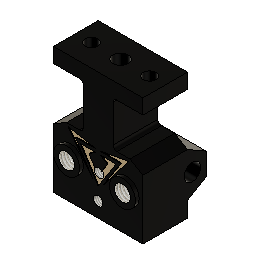
V2 Mothend (Autodesk Fusion 360 design; units mm, degrees)
part number: V2 Mothend BETA
Autodesk Fusion 360 part; units mm, degrees
ref_plane "WorkPlane1" through (0, 0, 3.5) normal (0, 0, 1) x (1, 0, 0) in component "Mothblock"
sketch "Sketch1" plane through (0, 0, 3.5) normal (0, 0, 1) x (0, 1, 0) in component "Mothblock"
  circle A0 centre (0, 0) radius 3.5
  line L0 (6, -12) -> (-6, -12)
  line L1 (-6, -12) -> (-6, 12)
  line L2 (-6, 12) -> (6, 12)
  line L3 (6, 12) -> (6, -12)
  line L4 (6, -12) -> (-6, 12) construction
  line L5 (-6, -12) -> (6, 12) construction
  line L6 (0, 7) -> (0, -7) construction
  line L7 (-3.75, 7.5) -> (3.75, 7.5) construction
  line L8 (3.75, 7.5) -> (3.75, -7.5) construction
  line L9 (3.75, -7.5) -> (-3.75, -7.5) construction
  line L10 (-3.75, -7.5) -> (-3.75, 7.5) construction
  line L11 (-3.75, 7.5) -> (3.75, -7.5) construction
  line L12 (3.75, 7.5) -> (-3.75, -7.5) construction
  dimension "d90" = 7
  dimension "d346" = 12
  dimension "d347" = 24
  dimension "d350" = 14
  dimension "d563" = 15
  dimension "d564" = 7.5
  constraint coincident A0.centre origin
  constraint horizontal L0
  constraint perpendicular L0 L1
  constraint parallel L0 L2
  constraint parallel L1 L3
  constraint coincident L4 A0.centre
  constraint coincident L5 A0.centre
  constraint vertical L6
  constraint midpoint A0.centre L6
  constraint horizontal L7
  constraint perpendicular L7 L8
  constraint parallel L7 L9
  constraint parallel L8 L10
  constraint coincident L11 A0.centre
  constraint coincident L12 A0.centre
  measures "d90" diameter of A0
  measures "d346" distance of L1.end L2.end
  measures "d347" distance of L0.end L1.end
  measures "d350" distance of L6.start L6.end
  measures "d563" distance of L7.end L8.end
  measures "d564" distance of L7.start L7.end
extrude "Extrude1" add sketch "Sketch1" along normal blind 34 contours A0 | L0 L1 L2 L3 in component "Mothblock"
hole "Hole8" [suppressed] in component "Mothblock"
thread "Thread9" [suppressed] in component "Mothblock"
hole "Hole15" at (-7.5, 3.75, 3.5) at (-7.5, -3.75, 3.5) at (7.5, 3.75, 3.5) at (7.5, -3.75, 3.5) direction (0, 0, 1) diameter 2.45 depth 6 tip angle 118 in component "Mothblock"
hole "Hole21" at (0, 0, 3.5) direction (0, 0, 1) diameter 4.1 end through all counterbore diameter 7.15 counterbore depth 14.5 in component "Mothblock"
sketch "Sketch7" plane through (0, -6, 0) normal (0, -1, 0) x (1, 0, 0) in component "Mothblock"
  line L0 (0, 3.5) -> (0, 37.5)
  line L1 (-12, 19.5) -> (-4, 24.1188)
  line L2 (-4, 24.1188) -> (-4, 33.5)
  line L3 (-12, 3.5) -> (12, 3.5)
  line L4 (12, 3.5) -> (12, 37.5)
  line L5 (12, 37.5) -> (-12, 37.5)
  line L6 (-12, 37.5) -> (-12, 3.5)
  line L7 (-4, 33.5) -> (-12, 33.5)
  line L8 (12, 19.5) -> (4, 24.1188)
  line L9 (4, 24.1188) -> (4, 33.5)
  line L10 (4, 33.5) -> (12, 33.5)
  line L11 (-8.5, 21.5207) -> (-4, 21.5207)
  line L12 (-4, 21.5207) -> (-4, 24.1188)
  line L13 (8.5, 21.5207) -> (4, 21.5207)
  line L14 (4, 21.5207) -> (4, 24.1188)
  line L15 (-6.25, 21.5207) -> (-4, 22.8198)
  line L16 (6.25, 21.5207) -> (4, 22.8198)
  dimension "d403" = 4
  dimension "d404" = 16
  dimension "d405" = 60
  dimension "d406" = 8
  dimension "d408" = 8
  dimension "d594" = 3.5
  dimension "d616" = 8
  dimension "d617" = 4.5
  dimension "d650" = 11.9793
  constraint vertical L0
  constraint symmetric L0 L1.start L8.start
  constraint symmetric L0 L1.end L8.end
  constraint symmetric L0 L2.end L9.end
  constraint symmetric L0 L7.end L10.end
  constraint coincident L6 L7.end
  constraint coincident L1.start L6
  constraint midpoint L0.start L3
  constraint horizontal L7
  constraint perpendicular L9 L10
  constraint midpoint L0.end L5
  constraint perpendicular L0 L11
  constraint coincident L1.end L2.start
  constraint perpendicular L11 L12
  constraint symmetric L0 L11.start L13.start
  constraint symmetric L0 L11.end L13.end
  constraint coincident L1 L11.start
  constraint midpoint L11 L15.start
  constraint coincident L12 L15.end
  constraint parallel L1 L15
  constraint symmetric L0 L15.start L16.start
  constraint symmetric L0 L15.end L16.end
  measures "d403" distance of L5.end L7.end
  measures "d404" distance of L1.start L3.start
  measures "d405" angle of L1 L6
  measures "d406" distance of L2 L9
  measures "d408" distance of L9.end L10.end
  measures "d594" horizontal distance of L1.start L11.start
  measures "d616" distance of L2.end L7.end
  measures "d617" distance of L11.start L11.end
  measures "d650" distance of L7 L11.start
extrude "Extrude7" cut sketch "Sketch7" against normal through all contours L1 L2 L6 L7 | L4 L8 L9 L10 | L1 L11 L12 L15 | L8 L13 L14 L16 | L11 L12 L15 | L13 L14 L16 in component "Mothblock"
sketch "Sketch2" plane through (0, 0, 37.5) normal (0, 0, 1) x (1, 0, 0) in component "Mothblock"
  circle A0 centre (0, 0) radius 2.05
  circle A1 centre (7.8, 0) radius 1.6
  circle A2 centre (-7.8, 0) radius 1.6
  line L0 (-7.8, 0) -> (7.8, 0) construction
  line L1 (-12, 6) -> (-12, -6)
  line L2 (-12, -6) -> (12, -6)
  line L3 (12, -6) -> (12, 6)
  line L4 (12, 6) -> (-12, 6)
  line L5 (-12, 6) -> (-4, 6)
  line L6 (-4, 6) -> (-4, -6)
  line L7 (-4, -6) -> (-12, -6)
  line L8 (-12, -6) -> (-12, 6)
  line L9 (-7.8, 6) -> (-7.8, -6) construction
  circle A3 centre (0, 0) radius 2.05
  dimension "d71" = 4.1
  dimension "d72" = 3.2
  dimension "d73" = 15.6
  constraint coincident A2.centre L0.start
  constraint coincident A1.centre L0.end
  constraint midpoint A0.centre L0
  constraint equal A1 A2
  constraint coincident A0.centre A3.centre
  constraint horizontal L0
  constraint coincident A2.centre L9
  constraint coincident L2 L9.end
  constraint coincident L4 L9.start
  constraint perpendicular L5 L9
  measures "d71" diameter of A0
  measures "d72" diameter of A1
  measures "d73" distance of A1.centre A2.centre
hole "Hole14" at (-7.8, 0, 37.5) at (7.8, 0, 37.5) direction (0, 0, -1) diameter 3.4 end up to surface (4 mm away) in component "Mothblock"
fillet "Fillet1" radius 1 4 edges at (4, 0, 21.5207) (-4, 0, 21.5207) (4, 0, 33.5) (-4, 0, 33.5) in component "Mothblock"
sketch "Sketch3" plane through (12, 0, 0) normal (-1, 0, 0) x (0, 1, 0) in component "Mothblock"
  line L0 (11, -16.6132) -> (11, -10.6132)
  line L1 (0, -3.5) -> (0, -19.5) construction
  line L2 (11, -16.6132) -> (6, -19.5)
  line L3 (11, -13.6132) -> (6, -13.6132) construction
  circle A0 centre (7.3175, -13.6132) radius 2.2425 construction
  line L4 (11, -10.6132) -> (6, -7.7265)
  line L5 (-3.5, -3.5) -> (3.5, -3.5)
  line L6 (6, -19.5) -> (-6, -19.5) construction
  line L7 (-6, -19.5) -> (-6, -3.5) construction
  line L8 (-6, -3.5) -> (6, -3.5) construction
  line L9 (6, -3.5) -> (6, -19.5) construction
  line L10 (-3.575, -3.5) -> (3.575, -3.5)
  line L11 (-3.575, -18) -> (3.575, -18)
  line L12 (3.575, -18) -> (3.575, -3.5) construction
  line L13 (6, -19.5) -> (6, -7.7265)
  dimension "d145" = 6
  dimension "d415" = 4.485
  dimension "d573" = 5
  dimension "d574" = 60
  dimension "d575" = 1.5
  dimension "d626" = 1.44
  dimension "d644" = 13.3175
  dimension "d645" = 10.1132
  constraint vertical L0
  constraint midpoint L0 L3.start
  constraint coincident L3 A0.centre
  constraint symmetric L0.start L3 L0.end
  constraint symmetric L3 L4.end L2.end
  constraint midpoint L1.end L6
  constraint midpoint L1.start L5
  constraint coincident L3.end L9
  constraint coincident L2.end L6.start
  constraint coincident L4.end L9
  constraint perpendicular L3 L9
  constraint coincident L11.end L12.start
  constraint coincident L10.end L12.end
  measures "d145" distance of L0.start L0.end
  measures "d415" diameter of A0
  measures "d573" horizontal distance of L3.start L3.end
  measures "d574" angle of L4 L9
  measures "d575" distance of A0 L12
  measures "d626" distance of L0 A0
  measures "d644" horizontal distance of A0.centre L7.end
  measures "d645" vertical distance of A0.centre L8.end
extrude "Extrude11" add sketch "Sketch3" along normal up to surface (24 mm away) in component "Mothblock"
hole "Hole13" at (12, 7.3175, 13.6132) direction (-1, 0, 0) diameter 4.4 depth 22 tip angle 180 in component "Mothblock"
sketch "Sketch16" plane through (12, 0, 0) normal (1, 0, 0) x (0, 1, 0) in component "Mothblock"
  circle A0 centre (7.3175, 13.6132) radius 2.2
  line L0 (6, 19.5) -> (-6, 19.5)
  line L1 (-6, 19.5) -> (-6, 3.5)
  line L2 (-6, 3.5) -> (6, 3.5)
  line L3 (6, 3.5) -> (6, 7.7265)
  line L4 (6, 7.7265) -> (11, 10.6132)
  line L5 (11, 10.6132) -> (11, 16.6132)
  line L6 (11, 16.6132) -> (6, 19.5)
  circle A1 centre (7.3175, 13.6132) radius 2.2
hole "Hole22" at (12, 7.3175, 13.6132) direction (-1, 0, 0) diameter 4.485 depth 3 tip angle 118 in component "Mothblock"
sketch "Sketch10" plane through (0, -6, 0) normal (0, 1, 0) x (-1, 0, 0) in component "Mothblock"
  line L0 (0, 0) -> (0, 3.5)
  line L1 (10, 13.6132) -> (0, 13.6132) construction
  line L2 (-3.575, 18) -> (-3.575, 3.5) construction
  line L3 (3.5, 27.2) -> (3.5, 14.2) construction
  line L4 (10, 15.8132) -> (-12, 15.8132) construction
  line L5 (10, 11.4132) -> (-12, 11.4132) construction
  circle A0 centre (-7.5, 13.6132) radius 2.5
  circle A1 centre (7.5, 13.6132) radius 2.5
  line L6 (-6.3895, 3.5) -> (-7.6105, 3.5)
  circle A2 centre (0, 14) radius 1.5
  circle A3 centre (0, 7.5) radius 1.5
  line L7 (-6.3895, 9.5) -> (-7.6105, 9.5)
  line L8 (-6.3, 3.5) -> (-8.7, 3.5)
  line L9 (-6.3, 9.5) -> (-8.7, 9.5)
  line L10 (12, 33.5) -> (5, 33.5)
  line L11 (4, 32.5) -> (4, 22.5207)
  line L12 (5, 21.5207) -> (8.5, 21.5207)
  line L13 (8.5, 21.5207) -> (12, 19.5)
  line L14 (12, 19.5) -> (12, 3.5)
  line L15 (12, 3.5) -> (-12, 3.5)
  line L16 (-12, 3.5) -> (-12, 19.5)
  line L17 (-12, 19.5) -> (-8.5, 21.5207)
  line L18 (-8.5, 21.5207) -> (-5, 21.5207)
  line L19 (-4, 22.5207) -> (-4, 32.5)
  line L20 (-5, 33.5) -> (-12, 33.5)
  line L21 (-12, 33.5) -> (-12, 37.5)
  line L22 (-12, 37.5) -> (12, 37.5)
  line L23 (12, 37.5) -> (12, 33.5)
  line L24 (10, 11.4132) -> (10, 15.8132)
  line L25 (3.575, 3.5) -> (-3.575, 3.5)
  line L26 (3.575, 18) -> (-3.575, 18)
  line L27 (-3.575, 10.75) -> (4.0823, 10.75) construction
  arc A4 (5, 33.5) -> (4, 32.5) centre (5, 32.5) ccw
  arc A5 (4, 22.5207) -> (5, 21.5207) centre (5, 22.5207) ccw
  arc A6 (-5, 21.5207) -> (-4, 22.5207) centre (-5, 22.5207) ccw
  arc A7 (-4, 32.5) -> (-5, 33.5) centre (-5, 32.5) ccw
  line L28 (-8.9745, 15.8132) -> (-8.9745, 11.4132)
  dimension "d370" = 5
  dimension "d371" = 15
  dimension "d383" = 3
  dimension "d385" = 3
  dimension "d429" = 1.5
  dimension "d593" = 4
  constraint coincident L0.start origin
  constraint coincident L0 L1.end
  constraint perpendicular L0 L1
  constraint symmetric L0 A0 A1
  constraint coincident L1 A0.centre
  constraint coincident L0 A2.centre
  constraint coincident L0 A3.centre
  constraint horizontal L4
  constraint horizontal L5
  constraint midpoint L1.start L24
  constraint coincident L2.start L26.end
  constraint coincident L2.end L15
  constraint coincident L2.end L25.end
  constraint coincident L4.start L24.end
  constraint coincident L5.start L24.start
  constraint midpoint L2 L27.start
  constraint perpendicular L2 L27
  constraint symmetric A2.centre A3.centre L27
  measures "d370" diameter of A0
  measures "d383" diameter of A2
  measures "d385" diameter of A3
  measures "d429" distance of L3 A1
  measures "d593" distance of A2.centre L26
hole "Hole17" at (7.5, -6, 13.6132) at (-7.5, -6, 13.6132) direction (0, 1, 0) diameter 4.234 depth 13.25 tip angle 180 in component "Mothblock"
thread "Thread20" "ISO Metric profile 5.0 M5x0.8 M5x0.8 6H" thread offset 0 thread depth 7.4 in component "Mothblock"
hole "Hole18" at (0, -6, 7.5) at (0, -6, 14) direction (0, 1, 0) diameter 2.529 depth 6 tip angle 180 in component "Mothblock"
thread "Thread17" "ISO Metric profile 3.0 M3x0.5 M3x0.5 6H" major diameter 3.086 minor diameter 2.529 pitch 0.5 angle 60 resizes the face on face at (-1.2645, -5.1146, 7.505) on face at (-1.2645, -5.1146, 14.005) in component "Mothblock"
sketch "Sketch12" plane through (0, -6, 0) normal (0, -1, 0) x (1, 0, 0) in component "Mothblock"
  circle A0 centre (0, 7.5) radius 1.2645
  circle A1 centre (0, 14) radius 1.2645
  circle A2 centre (7.5, 13.6132) radius 2.117
  circle A3 centre (-7.5, 13.6132) radius 2.117
  line L0 (-12, 33.5) -> (-5, 33.5)
  line L1 (-4, 32.5) -> (-4, 22.5207)
  line L2 (-5, 21.5207) -> (-8.5, 21.5207)
  line L3 (-8.5, 21.5207) -> (-12, 19.5)
  line L4 (-12, 19.5) -> (-12, 3.5)
  line L5 (-12, 3.5) -> (12, 3.5)
  line L6 (12, 3.5) -> (12, 19.5)
  line L7 (12, 19.5) -> (8.5, 21.5207)
  line L8 (8.5, 21.5207) -> (5, 21.5207)
  line L9 (4, 22.5207) -> (4, 32.5)
  line L10 (5, 33.5) -> (12, 33.5)
  line L11 (12, 33.5) -> (12, 37.5)
  line L12 (12, 37.5) -> (-12, 37.5)
  line L13 (-12, 37.5) -> (-12, 33.5)
  circle A4 centre (7.5, 13.6132) radius 2.117
  circle A5 centre (-7.5, 13.6132) radius 2.117
  circle A6 centre (7.5, 13.6132) radius 3.5
  circle A7 centre (-7.5, 13.6132) radius 3.5
  arc A8 (-4, 32.5) -> (-5, 33.5) centre (-5, 32.5) ccw
  arc A9 (-5, 21.5207) -> (-4, 22.5207) centre (-5, 22.5207) ccw
  arc A10 (4, 22.5207) -> (5, 21.5207) centre (5, 22.5207) ccw
  arc A11 (5, 33.5) -> (4, 32.5) centre (5, 32.5) ccw
  dimension "d624" = 7
  dimension "d625" = 1.383
  constraint equal A6 A7
  measures "d624" diameter of A6
  measures "d625" distance of A4 A6
extrude "Extrude20" add sketch "Sketch12" along normal blind 1 contours A6 | A7 in component "Mothblock"
sketch "Sketch14" plane through (0, -6, 0) normal (0, -1, 0) x (1, 0, 0) in component "Mothblock"
  spline S0 degree 3 poles (0.0304, 11.0848) (0.0854, 11.1563) (0.5074, 11.7942) (0.7506, 12.1736) knots 0 0 0 0 1 1 1 1
  spline S1 degree 3 poles (0.7506, 12.1736) (0.8585, 12.342) (1.1188, 12.749) (1.329, 13.0781) knots 0 0 0 0 1 1 1 1
  spline S2 degree 3 poles (1.329, 13.0781) (1.8478, 13.8905) (2.3833, 14.7224) (2.905, 15.5267) knots 0 0 0 0 1 1 1 1
  spline S3 degree 3 poles (2.905, 15.5267) (4.115, 17.3924) (4.6109, 18.1742) (4.6967, 18.3521) knots 0 0 0 0 1 1 1 1
  spline S4 degree 3 poles (4.6967, 18.3521) (4.7099, 18.3795) (4.7145, 18.3987) (4.709, 18.4042) knots 0 0 0 0 1 1 1 1
  spline S5 degree 3 poles (4.709, 18.4042) (4.6779, 18.4351) (3.4737, 18.479) (1.9183, 18.5058) knots 0 0 0 0 1 1 1 1
  spline S6 degree 3 poles (1.9183, 18.5058) (1.2764, 18.5169) (0.6185, 18.515) (0.6057, 18.5019) knots 0 0 0 0 1 1 1 1
  spline S7 degree 3 poles (0.6057, 18.5019) (0.5804, 18.4762) (0.8663, 18.2891) (1.6579, 17.8133) knots 0 0 0 0 1 1 1 1
  spline S8 degree 3 poles (1.6579, 17.8133) (2.2194, 17.4758) (2.4139, 17.3559) (2.4225, 17.342) knots 0 0 0 0 1 1 1 1
  spline S9 degree 3 poles (2.4225, 17.342) (2.4529, 17.2928) (2.2808, 17.0041) (1.626, 16.0063) knots 0 0 0 0 1 1 1 1
  spline S10 degree 3 poles (1.626, 16.0063) (1.2373, 15.4139) (0.8859, 14.8661) (0.4954, 14.2436) knots 0 0 0 0 1 1 1 1
  spline S11 degree 3 poles (0.4954, 14.2436) (0.2267, 13.8154) (0.1401, 13.687) (0.0731, 13.6176) knots 0 0 0 0 1 1 1 1
  spline S12 degree 3 poles (0.0731, 13.6176) (-0.0446, 13.4956) (-0.0998, 13.5241) (-0.2628, 13.7908) knots 0 0 0 0 1 1 1 1
  spline S13 degree 3 poles (-0.2628, 13.7908) (-0.4707, 14.131) (-0.9331, 14.855) (-1.494, 15.7185) knots 0 0 0 0 1 1 1 1
  spline S14 degree 3 poles (-1.494, 15.7185) (-1.9472, 16.4162) (-2.1645, 16.7582) (-2.3415, 17.0518) knots 0 0 0 0 1 1 1 1
  spline S15 degree 3 poles (-2.3415, 17.0518) (-2.4493, 17.2307) (-2.4791, 17.2878) (-2.473, 17.3037) knots 0 0 0 0 1 1 1 1
  spline S16 degree 3 poles (-2.473, 17.3037) (-2.4671, 17.3191) (-2.3512, 17.4068) (-2.2296, 17.4879) knots 0 0 0 0 1 1 1 1
  spline S17 degree 3 poles (-2.2296, 17.4879) (-2.0726, 17.5927) (-1.9073, 17.6951) (-1.5215, 17.9268) knots 0 0 0 0 1 1 1 1
  spline S18 degree 3 poles (-1.5215, 17.9268) (-0.9638, 18.2619) (-0.6582, 18.4568) (-0.6582, 18.4775) knots 0 0 0 0 1 1 1 1
  spline S19 degree 3 poles (-0.6582, 18.4775) (-0.6582, 18.497) (-0.8151, 18.5005) (-1.6403, 18.4998) knots 0 0 0 0 1 1 1 1
  spline S20 degree 3 poles (-1.6403, 18.4998) (-3.3283, 18.4983) (-4.7625, 18.4482) (-4.7849, 18.3899) knots 0 0 0 0 1 1 1 1
  spline S21 degree 3 poles (-4.7849, 18.3899) (-4.793, 18.3688) (-4.6567, 18.1524) (-3.7783, 16.7921) knots 0 0 0 0 1 1 1 1
  spline S22 degree 3 poles (-3.7783, 16.7921) (-3.4928, 16.3499) (-2.8563, 15.3611) (-2.3638, 14.5948) knots 0 0 0 0 1 1 1 1
  spline S23 degree 3 poles (-2.3638, 14.5948) (-0.9899, 12.4567) (-0.6801, 11.978) (-0.3264, 11.4473) knots 0 0 0 0 1 1 1 1
  spline S24 degree 3 poles (-0.3264, 11.4473) (-0.0802, 11.0779) (-0.047, 11.0316) (-0.0276, 11.0316) knots 0 0 0 0 1 1 1 1
  spline S25 degree 3 poles (-0.0276, 11.0316) (-0.0176, 11.0316) (0.0064, 11.0536) (0.0304, 11.0848) knots 0 0 0 0 1 1 1 1
  spline S26 degree 3 poles (1.4955, 12.0343) (1.6947, 12.2609) (1.9877, 12.6415) (2.8984, 13.8565) knots 0 0 0 0 1 1 1 1
  spline S27 degree 3 poles (2.8984, 13.8565) (3.3327, 14.4359) (3.9816, 15.2988) (4.3404, 15.7741) knots 0 0 0 0 1 1 1 1
  spline S28 degree 3 poles (4.3404, 15.7741) (4.6991, 16.2494) (5.2378, 16.9648) (5.5373, 17.3639) knots 0 0 0 0 1 1 1 1
  spline S29 degree 3 poles (5.5373, 17.3639) (6.2427, 18.3035) (6.5669, 18.732) (7.2084, 19.5722) knots 0 0 0 0 1 1 1 1
  spline S30 degree 3 poles (7.2084, 19.5722) (7.878, 20.4493) (8.0665, 20.6979) (8.0781, 20.7196) knots 0 0 0 0 1 1 1 1
  spline S31 degree 3 poles (8.0781, 20.7196) (8.0871, 20.7364) (8.0838, 20.7368) (7.979, 20.7304) knots 0 0 0 0 1 1 1 1
  spline S32 degree 3 poles (7.979, 20.7304) (7.8207, 20.7207) (7.4765, 20.664) (6.1165, 20.4237) knots 0 0 0 0 1 1 1 1
  spline S33 degree 3 poles (6.1165, 20.4237) (3.7034, 19.9972) (1.5433, 19.594) (0.8539, 19.4412) knots 0 0 0 0 1 1 1 1
  spline S34 degree 3 poles (0.8539, 19.4412) (0.6378, 19.3933) (0.6027, 19.3838) (0.6027, 19.3738) knots 0 0 0 0 1 1 1 1
  spline S35 degree 3 poles (0.6027, 19.3738) (0.6027, 19.3616) (0.6902, 19.3554) (1.0001, 19.3455) knots 0 0 0 0 1 1 1 1
  spline S36 degree 3 poles (1.0001, 19.3455) (1.3548, 19.3341) (3.0003, 19.3188) (3.91, 19.3184) knots 0 0 0 0 1 1 1 1
  spline S37 degree 3 poles (3.91, 19.3184) (4.8797, 19.318) (6.0012, 19.295) (6.0568, 19.2745) knots 0 0 0 0 1 1 1 1
  spline S38 degree 3 poles (6.0568, 19.2745) (6.0742, 19.268) (6.0742, 19.2674) (6.0568, 19.2286) knots 0 0 0 0 1 1 1 1
  spline S39 degree 3 poles (6.0568, 19.2286) (6.0471, 19.207) (5.9678, 19.0816) (5.8805, 18.95) knots 0 0 0 0 1 1 1 1
  spline S40 degree 3 poles (5.8805, 18.95) (5.7932, 18.8184) (5.578, 18.4866) (5.4022, 18.2128) knots 0 0 0 0 1 1 1 1
  spline S41 degree 3 poles (5.4022, 18.2128) (4.2765, 16.4585) (4.0506, 16.1081) (3.1015, 14.645) knots 0 0 0 0 1 1 1 1
  spline S42 degree 3 poles (3.1015, 14.645) (2.0136, 12.968) (1.4249, 12.0339) (1.4249, 11.9847) knots 0 0 0 0 1 1 1 1
  spline S43 degree 3 poles (1.4249, 11.9847) (1.4249, 11.9614) (1.4419, 11.9733) (1.4955, 12.0343) knots 0 0 0 0 1 1 1 1
  spline S44 degree 3 poles (-1.4713, 11.9943) (-1.4713, 12.0431) (-1.5797, 12.2281) (-1.809, 12.5711) knots 0 0 0 0 1 1 1 1
  spline S45 degree 3 poles (-1.809, 12.5711) (-2.5501, 13.6791) (-5.614, 18.4337) (-6.0384, 19.1343) knots 0 0 0 0 1 1 1 1
  spline S46 degree 3 poles (-6.0384, 19.1343) (-6.07, 19.1864) (-6.0924, 19.2322) (-6.0882, 19.236) knots 0 0 0 0 1 1 1 1
  spline S47 degree 3 poles (-6.0882, 19.236) (-6.0266, 19.2924) (-5.396, 19.3177) (-4.034, 19.3183) knots 0 0 0 0 1 1 1 1
  spline S48 degree 3 poles (-4.034, 19.3183) (-3.0662, 19.3188) (-1.4226, 19.3338) (-1.051, 19.3455) knots 0 0 0 0 1 1 1 1
  spline S49 degree 3 poles (-1.051, 19.3455) (-0.7416, 19.3552) (-0.6582, 19.3611) (-0.6582, 19.3733) knots 0 0 0 0 1 1 1 1
  spline S50 degree 3 poles (-0.6582, 19.3733) (-0.6582, 19.3873) (-0.9987, 19.4576) (-1.8916, 19.628) knots 0 0 0 0 1 1 1 1
  spline S51 degree 3 poles (-1.8916, 19.628) (-4.2817, 20.0841) (-7.8943, 20.7344) (-8.0377, 20.7344) knots 0 0 0 0 1 1 1 1
  line L0 (-8.0377, 20.7344) -> (-8.1043, 20.7344)
  line L1 (-8.1043, 20.7344) -> (-8.1043, 20.7091)
  spline S52 degree 3 poles (-8.1043, 20.7091) (-8.1043, 20.6952) (-8.0932, 20.6676) (-8.0797, 20.6477) knots 0 0 0 0 1 1 1 1
  spline S53 degree 3 poles (-8.0797, 20.6477) (-8.052, 20.6069) (-7.0395, 19.2675) (-6.2804, 18.2676) knots 0 0 0 0 1 1 1 1
  spline S54 degree 3 poles (-6.2804, 18.2676) (-5.4592, 17.1858) (-4.7582, 16.2563) (-3.6002, 14.7135) knots 0 0 0 0 1 1 1 1
  spline S55 degree 3 poles (-3.6002, 14.7135) (-2.3247, 13.0142) (-2.0778, 12.6899) (-1.747, 12.2787) knots 0 0 0 0 1 1 1 1
  spline S56 degree 3 poles (-1.747, 12.2787) (-1.532, 12.0115) (-1.4713, 11.9489) (-1.4713, 11.9943) knots 0 0 0 0 1 1 1 1
extrude "Extrude21" cut sketch "Sketch14" against normal blind 0.2 in component "Mothblock"
sketch "Sketch15" plane through (12, 0, 0) normal (1, 0, 0) x (0, 1, 0) in component "Mothblock"
  line L0 (6, 19.5) -> (-6, 19.5)
  line L1 (-6, 19.5) -> (-6, 3.5)
  line L2 (-6, 3.5) -> (6, 3.5)
  line L3 (6, 3.5) -> (6, 7.7265)
  line L4 (6, 7.7265) -> (11, 10.6132)
  line L5 (11, 10.6132) -> (11, 16.6132)
  line L6 (11, 16.6132) -> (6, 19.5)
  circle A0 centre (7.3175, 13.6132) radius 2.2425
component "Mothblock" placed x (1, 0, 0) y (0, 1, 0) z (0, 0, 1) at (0, 0, 0)
equation "d63 = mothblock_height"
equation "d347 = mothblock_width"
equation "d361 = mothblock_width - 2 mm"
equation "d415 = waterchannel_dia"
equation "d450 = coldend_length + 1 mm"
equation "mothblock_height = 34 mm"
equation "coldend_length = 13.5 mm"
equation "heatbreak_thread = 5.5 mm"
equation "heatbreak = 1.5 mm"
equation "waterchannel_dia = ballsize - 0.015 mm"
equation "ballsize = 4.5 mm"
equation "mothblock_width = 24 mm"
equation "d652 = waterchannel_dia"
named bodies: "Mothblock"
